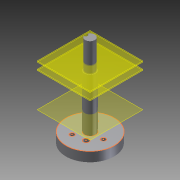
# Autodesk Inventor part: Jig_TopHeightAligner
Saved by Autodesk Inventor 2011 SP2 (Build 150309200, 309)
## iProperties
Created: 2011-09-29
Part Number: Jig_TopHeightAligner
Document SubType Name: Modeling
Designer: sungwook
Density: 1 g/cm^3
Author: sungwook
Autodesk Inventor part; units mm, degrees
ref_plane "YZ Plane" through (0, 0, 0) normal (1, 0, 0) x (0, 1, 0)
ref_plane "XZ Plane" through (0, 0, 0) normal (0, 1, 0) x (-1, 0, 0)
ref_plane "XY Plane" through (0, 0, 0) normal (0, 0, 1) x (1, 0, 0)
sketch "Sketch1" plane through (0, 0, 0) normal (0, 0, 1) x (1, 0, 0)
  circle A0 centre (0, 0) radius 12.7
  dimension "d0" = 25.4
  constraints: 1 centre point, 1 coincident
  measures "d0" diameter of A0
extrude "Extrusion1" add sketch "Sketch1" along normal blind 48.26
sketch "Sketch2" plane through (0, 0, 48.26) normal (0, 0, 1) x (1, 0, 0)
  circle A0 centre (0, 0) radius 12.7 projected
  circle A1 centre (0, 0) radius 2.9464
  dimension "d3" = 5.8928
  constraints: 1 centre point, 1 coincident
  measures "d3" diameter of A1
extrude "Extrusion2" cut sketch "Sketch2" against normal blind 43.18
sketch "Sketch3" plane through (0, 0, 0) normal (0, 0, -1) x (-1, 0, 0)
  circle A0 centre (-7, 0) radius 0.847
  circle A1 centre (3.5, 6.0622) radius 0.847
  arc A2 (5.3333, -1.3437) -> (5.3333, 1.3437) centre (6, 0) ccw
  circle A3 centre (3.5, -6.0622) radius 0.847
  circle A4 centre (6, 0) radius 1.5
  constraints: 5 centre point, 2 point on circle
hole "Hole1" at (7, 0, 0) at (-3.5, -6.0622, 0) at (-3.5, 6.0622, 0) direction (0, 0, 1) diameter 2.4384 end through all counterbore diameter 5.08 counterbore depth 2 clearance for "Flat Head Machine Screw (82)" size "#2" standard "Ansi Unified Screw Threads"
sketch "Sketch4" plane through (0, 0, 0) normal (0, 0, -1) x (-1, 0, 0)
  circle A0 centre (0, 0) radius 12.7 projected
  line L0 (0, 0) -> (-2.921, -5.0593)
  line L1 (0, -17.78) -> (0, 17.78) projected
  line L2 (17.78, 0) -> (-17.78, 0) projected
  dimension "d37" = 60
  dimension "d38" = 5.842
  constraints: 2 end point
  measures "d37" angle of L0 L2
  measures "d38" distance of L0.end L0.start
hole "Hole2" at (2.921, -5.0593, 0) direction (0, 0, 1) diameter 2.9972 end through all
sketch "Sketch5" plane through (0, 0, 5.08) normal (0, 0, 1) x (1, 0, 0)
  circle A0 centre (-3.5, 6.0622) radius 1.2192 projected
  circle A1 centre (-3.5, -6.0622) radius 1.2192 projected
  circle A2 centre (7, 0) radius 1.2192 projected
  circle A3 centre (0, 0) radius 2.9464 projected
  circle A4 centre (0, 0) radius 12.7 projected
  circle A5 centre (2.921, -5.0593) radius 1.4986 projected
ref_plane "Top Ref" through (0, 0, 37.4401) normal (0, 0, 1) x (1, 0, 0)
ref_plane "Bottom Ref" through (0, 0, 15.08) normal (0, 0, 1) x (1, 0, 0)
ref_plane "Work Plane4" through (0, 0, 33.6301) normal (0, 0, 1) x (1, 0, 0)
ref_plane "Work Plane5" through (0, 0, 33.1221) normal (0, 0, 1) x (1, 0, 0)
ref_plane "Work Plane6" through (0, 0, 36.9321) normal (0, 0, 1) x (1, 0, 0)
sketch "Sketch6" plane through (0, 0, 48.26) normal (0, 0, 1) x (1, 0, 0)
  circle A0 centre (0, 0) radius 2.9464 projected
  circle A1 centre (0, 0) radius 2.54
  dimension "d25" = 5.08
  constraints: 1 centre point, 1 coincident
  measures "d25" diameter of A1
extrude "Extrusion3" cut sketch "Sketch6" against normal up to surface (15.1379 mm away)
sketch "Sketch7" plane through (0, 0, 48.26) normal (0, 0, 1) x (1, 0, 0)
  circle A0 centre (0, 0) radius 2.54 projected
  circle A1 centre (-2.286, 0) radius 1.016
  dimension "d28" = 2.032
  dimension "d29" = 2.286
  constraints: 1 centre point, 1 horizontal alignment
  measures "d28" diameter of A1
  measures "d29" distance of A1.centre point (0, 0)
hole "Hole3" at (-2.286, 0, 48.26) direction (0, 0, -1) diameter 2.032 depth 11.3279
body "Solid1"
